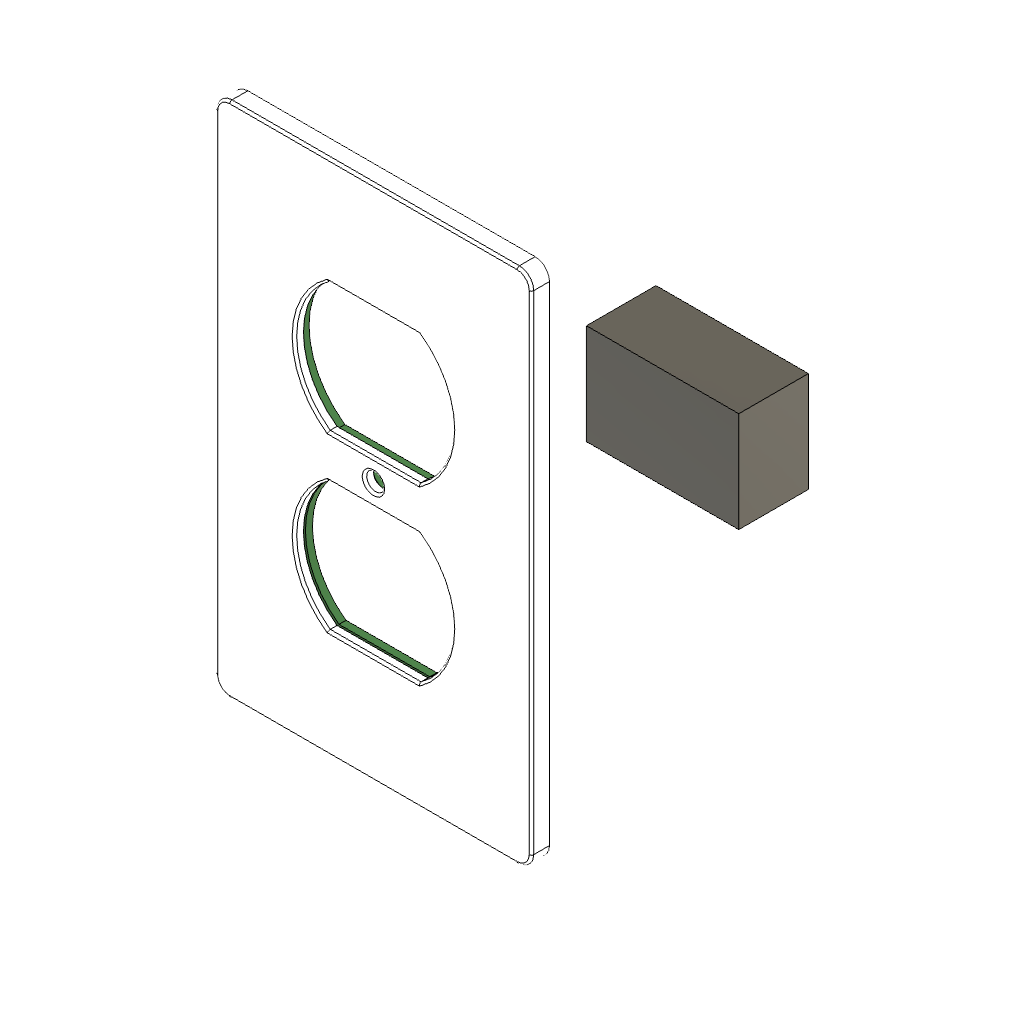
Wall Plate Model (Autodesk Fusion 360 design; units mm, degrees)
part number: 2026-09-17-10-58-23-669
Autodesk Fusion 360 part; units mm, degrees
sketch "Main shape" plane through (0, 0, 0) normal (0, 1, 0) x (1, 0, 0)
  line L0 (31.75, -57.15) -> (-31.75, -57.15)
  line L1 (-34.925, -53.975) -> (-34.925, 53.975)
  line L2 (-31.75, 57.15) -> (31.75, 57.15)
  line L3 (34.925, 53.975) -> (34.925, -53.975)
  line L4 (34.925, -57.15) -> (-34.925, 57.15) construction
  line L5 (-34.925, -57.15) -> (34.925, 57.15) construction
  circle A0 centre (0, 0) radius 1.984375
  circle A1 centre (0, -19.05) radius 17.4625
  arc A2 (-34.925, -53.975) -> (-31.75, -57.15) centre (-31.75, -53.975) ccw
  arc A3 (31.75, -57.15) -> (34.925, -53.975) centre (31.75, -53.975) ccw
  arc A4 (34.925, 53.975) -> (31.75, 57.15) centre (31.75, 53.975) ccw
  arc A5 (-31.75, 57.15) -> (-34.925, 53.975) centre (-31.75, 53.975) ccw
  line L6 (-10.040232, -4.7625) -> (10.040232, -4.7625)
  line L7 (-10.040232, -33.3375) -> (10.040232, -33.3375)
  line L8 (-34.925, 0) -> (34.925, 0) construction
  circle A6 centre (0, 19.05) radius 17.4625
  line L9 (-10.040232, 4.7625) -> (10.040232, 4.7625)
  line L10 (-10.040232, 33.3375) -> (10.040232, 33.3375)
  dimension "d1" = 69.85
  dimension "d2" = 114.3
  dimension "d3" = 3.96875
  dimension "d4" = 19.05
  dimension "d6" = 3.175
  dimension "d7" = 14.2875
  dimension "d8" = 14.2875
  dimension "d9" = 34.925
  constraint horizontal L0
  constraint perpendicular L0 L1
  constraint parallel L0 L2
  constraint parallel L1 L3
  constraint coincident L4 A0.centre
  constraint coincident L5 A0.centre
  constraint coincident A0.centre origin
  constraint coincident L5.start L0
  constraint coincident L5.start L1
  constraint tangent L0 A2
  constraint tangent L1 A2
  constraint coincident L4.start L0
  constraint coincident L4.start L3
  constraint tangent L0 A3
  constraint tangent L3 A3
  constraint equal A2 A3
  constraint coincident L5.end L3
  constraint coincident L5.end L2
  constraint tangent L3 A4
  constraint tangent L2 A4
  constraint equal A2 A4
  constraint coincident L4.end L1
  constraint coincident L4.end L2
  constraint tangent L1 A5
  constraint tangent L2 A5
  constraint equal A2 A5
  constraint horizontal L6
  constraint horizontal L7
  constraint midpoint L1 L8.start
  constraint midpoint L3 L8.end
  constraint symmetric A1 L8 A6
  measures "d1" distance of L4.end L5.end
  measures "d2" distance of L5.start L4.end
  measures "d3" diameter of A0
  measures "d4" distance of A0.centre A1.centre
  measures "d6" radius of A2
  measures "d7" distance of A1.centre L7
  measures "d8" distance of A1.centre L6
  measures "d9" diameter of A1
extrude "Extrude1" add sketch "Main shape" along normal blind 4 contours L0 L1 L2 L3 A2 A3 A4 A5 | A0 A6 L9 | A0 A1 L6 | A6 L10 | A1 L7 picked at (0.39587, -50.257356) picked at (-2.665914, 4.350543) picked at (0.044913, -3.834932) picked at (1.942864, 34.062019) picked at (-2.669498, -33.747609) makes body 1
fillet "Fillet1" radius 0.5 1 faces at (3.346744, 0, 49.2125) on bodies 1
sketch "Plate Cut-in" plane through (0, 4, 0) normal (0, 1, 0) x (-1, 0, 0)
  circle A0 centre (0, 0) radius 1.984375
  arc A1 (10.040232, 4.7625) -> (10.040232, 33.3375) centre (0, 19.05) ccw
  line L0 (10.040232, 4.7625) -> (-10.040232, 4.7625)
  arc A2 (-10.040232, 33.3375) -> (-10.040232, 4.7625) centre (0, 19.05) ccw
  line L1 (-10.040232, 33.3375) -> (10.040232, 33.3375)
  line L2 (-10.040232, -4.7625) -> (10.040232, -4.7625)
  arc A3 (10.040232, -33.3375) -> (10.040232, -4.7625) centre (0, -19.05) ccw
  line L3 (10.040232, -33.3375) -> (-10.040232, -33.3375)
  arc A4 (-10.040232, -4.7625) -> (-10.040232, -33.3375) centre (0, -19.05) ccw
  arc A5 (-34.925, -53.975) -> (-31.75, -57.15) centre (-31.75, -53.975) ccw
  line L4 (-31.75, -57.15) -> (31.75, -57.15)
  arc A6 (31.75, -57.15) -> (34.925, -53.975) centre (31.75, -53.975) ccw
  line L5 (34.925, -53.975) -> (34.925, 53.975)
  arc A7 (34.925, 53.975) -> (31.75, 57.15) centre (31.75, 53.975) ccw
  line L6 (31.75, 57.15) -> (-31.75, 57.15)
  arc A8 (-31.75, 57.15) -> (-34.925, 53.975) centre (-31.75, 53.975) ccw
  line L7 (-34.925, 53.975) -> (-34.925, -53.975)
  line L8 (-32.425, 53.975) -> (-32.425, -53.975)
  arc A9 (-32.425, -53.975) -> (-31.75, -54.65) centre (-31.75, -53.975) ccw
  line L9 (-31.75, -54.65) -> (31.75, -54.65)
  arc A10 (31.75, -54.65) -> (32.425, -53.975) centre (31.75, -53.975) ccw
  line L10 (32.425, -53.975) -> (32.425, 53.975)
  arc A11 (32.425, 53.975) -> (31.75, 54.65) centre (31.75, 53.975) ccw
  line L11 (31.75, 54.65) -> (-31.75, 54.65)
  arc A12 (-31.75, 54.65) -> (-32.425, 53.975) centre (-31.75, 53.975) ccw
  dimension "d14" = -2.5
extrude "Extrude2" cut sketch "Plate Cut-in" against normal blind 2 contours L8 A9 L9 A10 L10 A11 L11 A12 picked at (-3.346744, -47.545833) bodies 1
sketch "PCB" plane through (0, 4, 0) normal (0, 1, 0) x (-1, 0, 0)
  arc A0 (-34.925, -53.975) -> (-31.75, -57.15) centre (-31.75, -53.975) ccw
  line L0 (-31.75, -57.15) -> (31.75, -57.15)
  arc A1 (31.75, -57.15) -> (34.925, -53.975) centre (31.75, -53.975) ccw
  line L1 (34.925, -53.975) -> (34.925, 53.975)
  arc A2 (34.925, 53.975) -> (31.75, 57.15) centre (31.75, 53.975) ccw
  line L2 (31.75, 57.15) -> (-31.75, 57.15)
  arc A3 (-31.75, 57.15) -> (-34.925, 53.975) centre (-31.75, 53.975) ccw
  line L3 (-34.925, 53.975) -> (-34.925, -53.975)
  line L4 (-32.425, -53.975) -> (-32.425, 53.975)
  arc A4 (-31.75, 54.65) -> (-32.425, 53.975) centre (-31.75, 53.975) ccw
  line L5 (-31.75, 54.65) -> (31.75, 54.65)
  arc A5 (32.425, 53.975) -> (31.75, 54.65) centre (31.75, 53.975) ccw
  line L6 (32.425, 53.975) -> (32.425, -53.975)
  arc A6 (31.75, -54.65) -> (32.425, -53.975) centre (31.75, -53.975) ccw
  line L7 (31.75, -54.65) -> (-31.75, -54.65)
  arc A7 (-32.425, -53.975) -> (-31.75, -54.65) centre (-31.75, -53.975) ccw
  arc A8 (10.040232, 4.7625) -> (10.040232, 33.3375) centre (0, 19.05) ccw
  line L8 (10.040232, 4.7625) -> (-10.040232, 4.7625)
  arc A9 (-10.040232, 33.3375) -> (-10.040232, 4.7625) centre (0, 19.05) ccw
  line L9 (-10.040232, 33.3375) -> (10.040232, 33.3375)
  circle A10 centre (0, 0) radius 1.984375
  arc A11 (10.040232, -33.3375) -> (10.040232, -4.7625) centre (0, -19.05) ccw
  line L10 (10.040232, -33.3375) -> (-10.040232, -33.3375)
  arc A12 (-10.040232, -4.7625) -> (-10.040232, -33.3375) centre (0, -19.05) ccw
  line L11 (-10.040232, -4.7625) -> (10.040232, -4.7625)
  arc A13 (-31.75, 54.65) -> (-32.425, 53.975) centre (-31.75, 53.975) ccw
  line L12 (-32.425, 53.975) -> (-32.425, -53.975)
  arc A14 (-32.425, -53.975) -> (-31.75, -54.65) centre (-31.75, -53.975) ccw
  line L13 (-31.75, -54.65) -> (31.75, -54.65)
  arc A15 (31.75, -54.65) -> (32.425, -53.975) centre (31.75, -53.975) ccw
  line L14 (32.425, -53.975) -> (32.425, 53.975)
  arc A16 (32.425, 53.975) -> (31.75, 54.65) centre (31.75, 53.975) ccw
  line L15 (31.75, 54.65) -> (-31.75, 54.65)
  line L16 (-31.675, 53.9) -> (-31.675, -53.9)
  line L17 (-31.675, -53.9) -> (31.675, -53.9)
  line L18 (31.675, -53.9) -> (31.675, 53.9)
  line L19 (31.675, 53.9) -> (-31.675, 53.9)
  line L20 (10.274665, 4.0125) -> (-10.274665, 4.0125)
  arc A17 (-10.274665, 34.0875) -> (-10.274665, 4.0125) centre (0, 19.05) ccw
  line L21 (-10.274665, 34.0875) -> (10.274665, 34.0875)
  arc A18 (10.274665, 4.0125) -> (10.274665, 34.0875) centre (0, 19.05) ccw
  arc A19 (9.800191, -32.5875) -> (9.800191, -5.5125) centre (0, -19.05) ccw
  line L22 (-9.800191, -5.5125) -> (9.800191, -5.5125)
  arc A20 (-9.800191, -5.5125) -> (-9.800191, -32.5875) centre (0, -19.05) ccw
  line L23 (9.800191, -32.5875) -> (-9.800191, -32.5875)
  circle A21 centre (0, 0) radius 2.484375
  dimension "d17" = -0.75
  dimension "d18" = 0.75
  dimension "d19" = 0.75
  dimension "d20" = 0.5
extrude "Extrude3" add sketch "PCB" against normal blind 1.5748 separate body contours L16 L17 L18 L19 picked at (-3.346744, -47.045833) makes body 2
sketch "Sketch4" plane through (0, 4, 0) normal (0, 1, 0) x (-1, 0, 0)
  circle A0 centre (0, 0) radius 2.484375
  arc A1 (10.040232, -33.3375) -> (10.040232, -4.7625) centre (0, -19.05) ccw
  line L0 (10.040232, -33.3375) -> (-10.040232, -33.3375)
  arc A2 (-10.040232, -4.7625) -> (-10.040232, -33.3375) centre (0, -19.05) ccw
  line L1 (-10.040232, -4.7625) -> (10.040232, -4.7625)
  arc A3 (-10.274665, 34.0875) -> (-10.274665, 4.0125) centre (0, 19.05) ccw
  line L2 (-10.274665, 34.0875) -> (10.274665, 34.0875)
  arc A4 (10.274665, 4.0125) -> (10.274665, 34.0875) centre (0, 19.05) ccw
  line L3 (10.274665, 4.0125) -> (-10.274665, 4.0125)
  line L4 (31.675, 53.9) -> (-31.675, 53.9)
  line L5 (-31.675, 53.9) -> (-31.675, -53.9)
  line L6 (-31.675, -53.9) -> (31.675, -53.9)
  line L7 (31.675, -53.9) -> (31.675, 53.9)
  line L8 (-76.749143, 49.578151) -> (-43.049143, 49.578151)
  line L9 (-43.049143, 49.578151) -> (-43.049143, 27.378151)
  line L10 (-43.049143, 27.378151) -> (-76.749143, 27.378151)
  line L11 (-76.749143, 27.378151) -> (-76.749143, 49.578151)
  dimension "d23" = 33.7
  dimension "d24" = 22.2
  constraint horizontal L8
  constraint vertical L9
  constraint horizontal L10
  constraint vertical L11
extrude "Extrude4" add sketch "Sketch4" along normal blind 15.4 separate body contours L8 L9 L10 L11 picked at (-54.282477, 42.178151) makes body 3
named bodies: "Wall Plate", "PCB"
